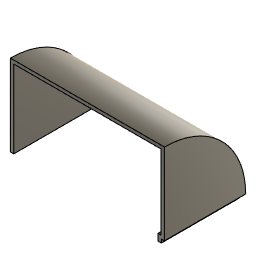
Vent Redirector v2 (Autodesk Fusion 360 design; units mm, degrees)
Autodesk Fusion 360 part; units mm, degrees
sketch "Sketch1" plane through (0, 0, 0) normal (0, 0, 1) x (1, 0, 0)
  line L0 (0, 0) -> (144.4625, 0)
  line L1 (144.4625, 0) -> (144.4625, -76.2)
  line L2 (0, -76.2) -> (0, 0)
  line L3 (0, -76.2) -> (3.175, -76.2)
  line L4 (144.4625, -76.2) -> (141.2875, -76.2)
  line L5 (3.175, -76.2) -> (3.175, -3.175)
  line L6 (141.2875, -76.2) -> (141.2875, -3.175)
  line L7 (3.175, -3.175) -> (141.2875, -3.175)
  dimension "d2" = 144.4625
  dimension "d3" = 76.2
  dimension "d5" = 3.175
  dimension "d6" = 3.175
  dimension "d7" = 73.025
  dimension "d8" = 73.025
  constraint horizontal L0
  constraint vertical L1
  constraint vertical L2
  constraint coincident L0.start L2.end
  constraint perpendicular L2 L3
  constraint perpendicular L1 L4
  constraint perpendicular L3 L5
  constraint perpendicular L4 L6
  constraint perpendicular L6 L7
  measures "d2" distance of L0.start L0.end
  measures "d3" distance of L0.start L2.start
  measures "d5" distance of L2.start L3.end
  measures "d6" distance of L1.end L4.end
  measures "d7" distance of L3.end L5.end
  measures "d8" distance of L4.end L6.end
revolve "Revolve1" add sketch "Sketch1" angle 90 about axis through (127, -76.2, 0) along (1, 0, 0) makes body 1
sketch "Sketch2" plane through (0, 0, 0) normal (0, 0, 1) x (1, 0, 0)
  line L0 (137.16, 0) -> (140.335, 0)
  line L1 (140.335, 0) -> (140.335, -73.025)
  line L2 (140.335, -73.025) -> (137.16, -73.025)
  line L3 (137.16, -73.025) -> (137.16, 0)
  dimension "d13" = 3.175
  dimension "d14" = 73.025
  constraint horizontal L0
  constraint vertical L1
  constraint horizontal L2
  constraint vertical L3
  measures "d13" distance of L0.start L0.end
  measures "d14" distance of L0.start L2.end
extrude "Extrude1" add sketch "Sketch2" along normal blind 3.175 separate body makes body 2
move_body "Move1" bodies 2 to x (1, 0, 0) y (0, 1, 0) z (0, 0, 1) at (1.27, -3.175, 0)
extrude "Extrude2" add 1 faces at (139.4883, -51.8583, 0) along direction (0, 0, -1) blind 3.175 on bodies 2 bodies 2 1
equation "d2 = Length"
equation "d3 = Width"
equation "d5 = Thicc"
equation "d6 = Thicc"
equation "d7 = Depth"
equation "d8 = Depth"
equation "Depth = 2.875 in"
equation "Length = 5.6875 in"
equation "Width = 3 in"
equation "Thicc = 0.125 in"
equation "d13 = Thicc"
equation "d15 = Thicc"
equation "d18 = Thicc"
